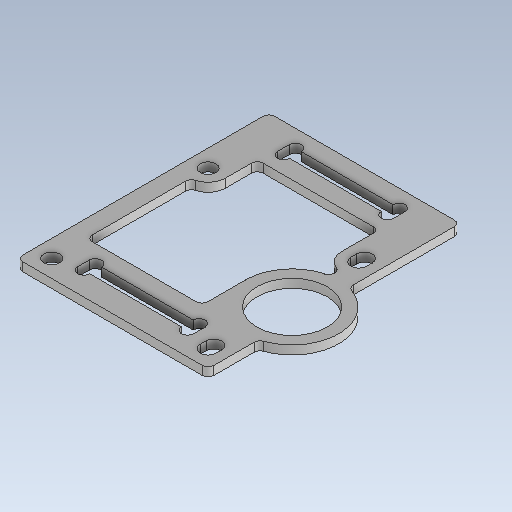
# Autodesk Inventor part: Trunk_vertical_frame_06
Saved by Autodesk Inventor 2020.4 (Build 244396000, 396)
## iProperties
Created: 2021-09-08
Part Number: Trunk_vertical_frame_06
Material: 一般
Document SubType Name: Modeling
Designer: Masato Kubotera
Density: 1 g/cm^3
Appearance: 既定
Mass: 1.05119 g
Surface Area: 20.3851 cm^2
Volume: 1.05119 cm^3
Description: A2017 T1.5
Author: moonk
Autodesk Inventor part; units mm, degrees
ref_plane "YZ Plane" through (0, 0, 0) normal (1, 0, 0) x (0, 1, 0)
ref_plane "XZ Plane" through (0, 0, 0) normal (0, 1, 0) x (-1, 0, 0)
ref_plane "XY Plane" through (0, 0, 0) normal (0, 0, 1) x (1, 0, 0)
sketch "スケッチ1" plane through (0, 0, 0) normal (0, 0, 1) x (1, 0, 0)
  circle A0 centre (0, 0) radius 6.05
  arc A1 (2, -7.7976) -> (2, 7.7976) centre (0, 0) ccw
  line L0 (-31, 0) -> (0, 0) construction
  line L1 (-24.51, 24.01) -> (-4.49, 24.01)
  line L2 (-4.49, 24.01) -> (-4.49, 21.99)
  line L3 (-4.49, 21.99) -> (-24.51, 21.99)
  line L4 (-24.51, 21.99) -> (-24.51, 24.01)
  line L5 (-24.51, 24.01) -> (-4.49, 21.99) construction
  line L6 (-4.49, 24.01) -> (-24.51, 21.99) construction
  line L7 (-24.5, 24) -> (-4.5, 24) construction
  line L8 (-4.5, 24) -> (-4.5, 22) construction
  line L9 (-4.5, 22) -> (-24.5, 22) construction
  line L10 (-24.5, 22) -> (-24.5, 24) construction
  line L11 (-24.5, 24) -> (-4.5, 22) construction
  line L12 (-4.5, 24) -> (-24.5, 22) construction
  line L13 (-24.51, 23) -> (-4.49, 23) construction
  arc A2 (-22.41, 24.01) -> (-24.51, 24.01) centre (-23.46, 24.01) ccw
  arc A3 (-24.51, 21.99) -> (-22.41, 21.99) centre (-23.46, 21.99) ccw
  line L14 (-14.5, 24) -> (-14.5, 21.99) construction
  arc A4 (-4.49, 24.01) -> (-6.59, 24.01) centre (-5.54, 24.01) ccw
  arc A5 (-6.59, 21.99) -> (-4.49, 21.99) centre (-5.54, 21.99) ccw
  line L15 (-28, 13.5) -> (-1, 13.5) construction
  line L16 (-1, 13.5) -> (-1, -13.5) construction
  line L17 (-1, -13.5) -> (-28, -13.5) construction
  line L18 (-28, -13.5) -> (-28, 13.5) construction
  line L19 (-28, 13.5) -> (-1, -13.5) construction
  line L20 (-1, 13.5) -> (-28, -13.5) construction
  line L21 (-14.5, 13.5) -> (-14.5, -13.5) construction
  line L22 (-24.51, -10.49) -> (-4.49, -10.49)
  line L23 (-4.49, -10.49) -> (-4.49, -12.51)
  line L24 (-4.49, -12.51) -> (-24.51, -12.51)
  line L25 (-24.51, -12.51) -> (-24.51, -10.49)
  line L26 (-24.51, -10.49) -> (-4.49, -12.51) construction
  line L27 (-4.49, -10.49) -> (-24.51, -12.51) construction
  line L28 (-24.5, -10.5) -> (-4.5, -10.5) construction
  line L29 (-4.5, -10.5) -> (-4.5, -12.5) construction
  line L30 (-4.5, -12.5) -> (-24.5, -12.5) construction
  line L31 (-24.5, -12.5) -> (-24.5, -10.5) construction
  line L32 (-24.5, -10.5) -> (-4.5, -12.5) construction
  line L33 (-4.5, -10.5) -> (-24.5, -12.5) construction
  line L34 (-24.51, -11.5) -> (-4.49, -11.5) construction
  arc A6 (-22.41, -10.49) -> (-24.51, -10.49) centre (-23.46, -10.49) ccw
  arc A7 (-24.51, -12.51) -> (-22.41, -12.51) centre (-23.46, -12.51) ccw
  line L35 (-14.5, -10.5) -> (-14.5, -12.51) construction
  arc A8 (-4.49, -10.49) -> (-6.59, -10.49) centre (-5.54, -10.49) ccw
  arc A9 (-6.59, -12.51) -> (-4.49, -12.51) centre (-5.54, -12.51) ccw
  line L36 (-31, 27) -> (-31, -16.5)
  line L37 (-31, -16.5) -> (2, -16.5)
  line L38 (2, -16.5) -> (2, -7.7976)
  line L39 (2, 7.7976) -> (2, 27)
  line L40 (2, 27) -> (-31, 27)
  arc A10 (-28, 10.5) -> (-25, 13.5) centre (-28, 13.5) ccw
  line L41 (-28, 10.5) -> (-28, 10.5)
  line L42 (-28, 10.5) -> (-28, -7.5)
  line L43 (-28, -7.5) -> (-8.05, -7.5)
  line L44 (-8.05, -7.5) -> (-8.05, 0)
  line L45 (-25, 13.5) -> (-25, 19)
  line L46 (-25, 19) -> (-4, 19)
  arc A11 (-1, 7.9876) -> (-8.05, 0) centre (0, 0) ccw
  line L47 (-1, 9.5) -> (-1, 7.9876)
  circle A12 centre (-28, 13.5) radius 1.35
  arc A13 (0.35, 13.5) -> (-2.35, 13.5) centre (-1, 13.5) ccw
  arc A14 (-2.35, 12.5) -> (0.35, 12.5) centre (-1, 12.5) ccw
  arc A15 (-4, 12.5) -> (-1, 9.5) centre (-1, 12.5) ccw
  line L48 (0.35, 12.5) -> (0.35, 13.5)
  line L49 (-2.35, 13.5) -> (-2.35, 12.5)
  line L50 (-4, 19) -> (-4, 12.5)
  arc A16 (-2.35, -13.5) -> (0.35, -13.5) centre (-1, -13.5) ccw
  arc A17 (0.35, -12.5) -> (-2.35, -12.5) centre (-1, -12.5) ccw
  line L51 (0.35, -12.5) -> (0.35, -13.5)
  line L52 (-2.35, -13.5) -> (-2.35, -12.5)
  circle A18 centre (-28, -13.5) radius 1.35
  point P0 (-14.5, 23)
  point P1 (-14.5, 0)
  point P2 (-14.5, -11.5)
  point P3 (-14.5, 22.995)
  point P4 (-6.59, -10.49)
  point P5 (-6.59, -12.51)
  point P6 (-22.41, -12.51)
  point P7 (-6.59, 24.01)
  dimension "d96" = 12.1
  dimension "d215" = 20
  dimension "d216" = 2
  dimension "d217" = 0.01
  dimension "d219" = 0.01
  dimension "d220" = 1.05
  dimension "d222" = 27
  dimension "d223" = 27
  dimension "d226" = 20
  dimension "d227" = 2
  dimension "d228" = 0.01
  dimension "d229" = 0.01
  dimension "d230" = 1.05
  dimension "d231" = 32.5
  dimension "d238" = 3
  dimension "d240" = 3
  dimension "d241" = 3
  dimension "d242" = 4
  dimension "d243" = 3
  dimension "d244" = 2
  dimension "d245" = 3
  dimension "d246" = 3
  dimension "d247" = 3
  dimension "d248" = 3
  dimension "d251" = 2
  dimension "d252" = 3
  dimension "d255" = 1
  dimension "d257" = 2.7
  dimension "d259" = 2.7
  dimension "d260" = 1
  dimension "d262" = 3
  constraints: 106 end point, 32 point on circle, 21 midpoint, 19 centre point, 19 symmetric about line, 16 point on line, 12 parallel, 10 perpendicular, 7 horizontal, 6 coincident, 6 vertical, 4 tangent, 1 collinear, 1 concentric, 9 other
  measures "d96" diameter of A0
  measures "d215" distance of L8.end L9.end
  measures "d216" distance of L7.end L8.end
  measures "d217" horizontal distance of L1.start L7.start
  measures "d219" horizontal distance of L7.start L1.start
  measures "d220" radius of A2
  measures "d222" distance of L16.end L17.end
  measures "d223" distance of L15.end L16.end
  measures "d226" distance of L30.start L31.start
  measures "d227" distance of L33.start L30.start
  measures "d228" horizontal distance of L25.end L31.end
  measures "d229" horizontal distance of L31.end L25.end
  measures "d230" radius of A6
  measures "d231" distance of L31.end L9.end
  measures "d238" vertical distance of L16.end L33.start
  measures "d240" horizontal distance of L36.end L17.end
  measures "d241" horizontal distance of L17.end L36.end
  measures "d242" vertical distance of L36.end L31.start
  measures "d243" vertical distance of L7.start L36.start
  measures "d244" radial gap between concentric circles of A1 A0
  measures "d245" horizontal distance of L36.start L41.end
  measures "d246" horizontal distance of L39.start L47.start
  measures "d247" vertical distance of L45.end L9.end
  measures "d248" distance of L45.start A10.centre
  measures "d251" radial gap between concentric circles of A11 A0
  measures "d252" distance from line of L31.end L43
  measures "d255" distance from line of L16 point (0, 0)
  measures "d257" diameter of A12
  measures "d259" diameter of A13
  measures "d260" distance of A14.centre L15.end
  measures "d262" horizontal distance of L46.end L15.end
extrude "押し出し1" add sketch "スケッチ1" along normal blind 1.5
fillet "フィレット1" radius 1 7 edges at (-1, 7.9876, 0.75) (-8.05, -7.5, 0.75) (-28, -7.5, 0.75) (-25, 19, 0.75) (-28, 10.5, 0.75) (-4, 19, 0.75) (-1, 9.5, 0.75)
fillet "フィレット2" radius 1 6 edges at (-31, 27, 0.75) (2, 27, 0.75) (-31, -16.5, 0.75) (2, -7.7976, 0.75) (2, -16.5, 0.75) (2, 7.7976, 0.75)
